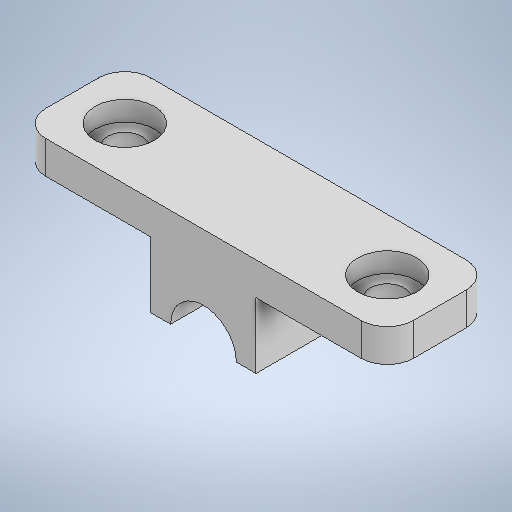
# Autodesk Inventor part: led_holder
Saved by Autodesk Inventor 2025 (Build 290162000, 162)
## iProperties
Created: 2026-05-12
Part Number: led_holder
Material: Ogólny
Document SubType Name: Modeling
Designer: zzapa
Density: 1 g/cm^3
Appearance: Domyślna
Author: zzapa
Autodesk Inventor part; units mm, degrees
ref_plane "YZ Plane" through (0, 0, 0) normal (1, 0, 0) x (0, 1, 0)
ref_plane "XZ Plane" through (0, 0, 0) normal (0, 1, 0) x (-1, 0, 0)
ref_plane "XY Plane" through (0, 0, 0) normal (0, 0, 1) x (1, 0, 0)
sketch "Szkic1" plane through (0, 0, 0) normal (0, 1, 0) x (-1, 0, 0)
  line L0 (28, 0) -> (0, 0)
  line L1 (0, 0) -> (0, -8)
  line L2 (0, -8) -> (28, -8)
  line L3 (28, -8) -> (28, 0)
  dimension "d0" = 8
  dimension "d4" = 28
  constraints: 8 end point, 2 parallel, 1 coincident, 1 horizontal, 1 perpendicular
  measures "d0" distance of L2.end L0.start
  measures "d4" distance of L1.end L2.end
extrude "Wyciągnięcie proste1" add sketch "Szkic1" along normal blind 2.5
sketch "Szkic2" plane through (0, 2.5, 0) normal (0, 1, 0) x (1, 0, 0)
  line L0 (-28, 0) -> (0, 0) projected
  line L1 (0, 8) -> (-28, 8) projected
  line L2 (-14, 0) -> (-14, 8)
  line L3 (-24, 4) -> (-4, 4)
  point P0 (-14, 4)
  dimension "d3" = 20
  constraints: 4 end point, 4 midpoint, 1 coincident, 1 horizontal, 1 symmetric about line
  measures "d3" distance of point (-4, 4) point (-24, 4)
hole "Otwór1" at (-24, 2.5, -4) at (-4, 2.5, -4) direction (0, -1, 0) diameter 2.6 end through all counterbore diameter 4.5 counterbore depth 1.5
sketch "Szkic3" plane through (-28, 0, 0) normal (0, 0, 1) x (1, 0, 0)
  line L0 (14, 2.5) -> (14, 0)
  line L1 (0, 2.5) -> (28, 2.5) projected
  line L2 (0, 0) -> (28, 0) projected
  circle A0 centre (14, -5) radius 2.5
  line L3 (10, -5) -> (18, -5)
  line L4 (18, -5) -> (18, 0)
  line L5 (10, 0) -> (10, -5)
  line L6 (18, 0) -> (10, 0)
  point P0 (10, 3)
  point P1 (17.6174, 3)
  point P2 (16.5, -5)
  point P3 (11.5, -5)
  point P4 (14, 0)
  point P5 (18, 0)
  dimension "d12" = 5
  dimension "d13" = 8
  dimension "d17" = 5
  constraints: 10 end point, 5 midpoint, 2 horizontal, 1 centre point, 1 coincident, 1 collinear, 1 parallel, 1 perpendicular, 1 vertical
  measures "d12" diameter of A0
  measures "d13" distance between parallel lines of L5 L4
  measures "d17" distance of L3.end L4.end
extrude "Wyciągnięcie proste2" add sketch "Szkic3" against normal up to surface (8 mm away) contours L2 L4 L3 A0 L5
fillet "Zaokrąglenie1" radius 2 4 edges at (0, 1.25, 0) (0, 1.25, -8) (-28, 1.25, -8) (-28, 1.25, 0)
equation "\"d0\" = obudowa_led_mocowanie_grubosc"
equation "\"d4\" = holder_led_dlugosc"
equation "\"d1\" = holder_led_grubosc"
equation "\"d3\" = obudowa_led_mocowanie_rozstaw_otworow"
equation "\"d5\" = gniazdo_M2_D2"
equation "\"d7\" = gniazdo_M2_D1"
equation "\"d8\" = gniazdo_M2_glebokosc"
equation "\"d10\" = insert_glebokosc"
equation "\"d12\" = holder_led_uchwyt_D"
equation "\"d13\" = holder_led_uchwyt_szerokosc"
equation "\"d17\" = holder_led_uchwyt_wysokosc"
equation "\"gniazdo_M2_glebokosc\" = 1.5"
equation "\"gniazdo_M2_D1\" = 4.5"
equation "\"gniazdo_M2_D2\" = 2.6"
equation "\"insert_D\" = 2.9"
equation "\"insert_glebokosc\" = 7"
equation "\"podstawa_wys\" = 2"
equation "\"podstawa_otwory_montazowe_poz_x\" = 4"
equation "\"podstawa_otwory_montazowe_poz_y\" = 4"
equation "\"podstawa_zaokraglenie\" = 3"
equation "\"obudowa_wys\" = 45"
equation "\"obudowa_grubosc\" = 2"
equation "\"obudowa_kontrolki_a\" = 38"
equation "\"obudowa_otwory_montazowe_poz_x\" = 4"
equation "\"obudowa_otwory_montazowe_poz_y\" = 4"
equation "\"obudowa_otwory_montazowe_material_x\" = 8"
equation "\"obudowa_otwory_montazowe_material_y\" = 8"
equation "\"obudowa_zaokraglenie\" = 3"
equation "\"obudowa_otwory_io1_D\" = 12"
equation "\"obudowa_otwory_io1_wys\" = 25"
equation "\"obudowa_otwory_io1_poz\" = 55"
equation "\"obudowa_otwory_io2_D\" = 12"
equation "\"obudowa_otwory_io2_wys\" = 25"
equation "\"obudowa_otwory_io2_poz\" = 38"
equation "\"obudowa_otwory_pot_D\" = 7.2"
equation "\"obudowa_pot_poz_y\" = 15"
equation "\"obudowa_s_rozstaw_y\" = 16"
equation "\"obudowa_s_poz_x\" = 78"
equation "\"obudowa_s_poz_y\" = 15"
equation "\"obudowa_s_D\" = 6.2"
equation "\"input_a\" = 8.9"
equation "\"input_b\" = 14.4"
equation "\"input_wys\" = 10.9"
equation "\"obudowa_MTS_otwor_D\" = 6.2"
equation "\"pcb_rozstaw_x\" = 92"
equation "\"pcb_rozstaw_y\" = 58"
equation "\"pcb_grubosc_scianki\" = 6"
equation "\"pcb_wys_bloku\" = 35"
equation "\"pcb_poz_y\" = 29"
equation "\"obudowa_footswitch_D\" = 12.3"
equation "\"obudowa_footswitch_poz_x\" = 35"
equation "\"obudowa_footswitch_poz_y\" = 68"
equation "\"obudowa_led_indicator_D\" = 3.5"
equation "\"obudowa_led_indicator_poz_x\" = 55"
equation "\"obudowa_podkladka_otwory\" = 4"
equation "\"obudowa_uchwyt_poz_z\" = 3"
equation "\"obudowa_uchwyt_grubosc\" = 2"
equation "\"obudowa_uchwyt_szerokosc_wew\" = 17.5"
equation "\"obudowa_uchwyt_wysokosc_wew\" = 26.3"
equation "\"obudowa_uchwyt_kolnierz_wys\" = 55"
equation "\"obudowa_gniazdo_poz\" = 25"
equation "\"obudowa_podciecie_inout_wys\" = 6"
equation "\"obudowa_podciecie_logo_wys\" = 34"
equation "\"obudowa_podciecie_logo_szerokosc\" = 25"
equation "\"obudowa_pot_pozycjonowanie_szerokosc\" = 2.8"
equation "\"obudowa_pot_pozycjonowanie_wys\" = 13"
equation "\"obudowa_pot_pozycjonowanie_glebokosc\" = 1.4"
equation "\"obudowa_led_mocowanie_wys\" = 6"
equation "\"obudowa_led_mocowanie_grubosc\" = 8"
equation "\"obudowa_led_mocowanie_rozstaw_otworow\" = 20"
equation "\"holder_led_grubosc\" = 2.5"
equation "\"holder_led_dlugosc\" = 28"
equation "\"holder_led_uchwyt_D\" = 5"
equation "\"holder_led_uchwyt_wysokosc\" = 5"
equation "\"holder_led_uchwyt_szerokosc\" = 8"
